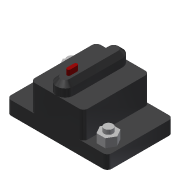
# Autodesk Inventor part: 120 Amp Breaker - Bussman
Saved by Autodesk Inventor 2013 (Build 170138000, 138)
## iProperties
Created: 2013-12-22
Part Number: 120 Amp Breaker - Bussman
Material: Generic
Document SubType Name: Modeling
Designer: Nemo
Mass: 108.862 g
Surface Area: 146.665 cm^2
Volume: 77.8352 cm^3
Density: 1.39862 g/cm^3
Author: Nemo
Autodesk Inventor part; units mm, degrees
ref_plane "YZ Plane" through (0, 0, 0) normal (1, 0, 0) x (0, 1, 0)
ref_plane "XZ Plane" through (0, 0, 0) normal (0, 1, 0) x (-1, 0, 0)
ref_plane "XY Plane" through (0, 0, 0) normal (0, 0, 1) x (1, 0, 0)
sketch "Sketch2" plane through (0, 0, 0) normal (0, 1, 0) x (-1, 0, 0)
  line L0 (36.83, -24.13) -> (-36.83, -24.13)
  line L1 (-36.83, -24.13) -> (-36.83, 24.13)
  line L2 (-36.83, 24.13) -> (36.83, 24.13)
  line L3 (36.83, 24.13) -> (36.83, -24.13)
  line L4 (36.83, -24.13) -> (-36.83, 24.13) construction
  line L5 (-36.83, -24.13) -> (36.83, 24.13) construction
  point P0 (0, 0)
  point P1 (0, 0)
  point P2 (0, 0)
  dimension "d2" = 73.66
  dimension "d3" = 48.26
  constraints: 12 end point, 3 midpoint, 2 parallel, 1 coincident, 1 horizontal, 1 perpendicular
  measures "d2" distance of L1.end L2.end
  measures "d3" distance of L0.end L1.end
extrude "Extrusion1" add sketch "Sketch2" along normal blind 9.906
sketch "Sketch3" plane through (0, 9.906, 0) normal (0, 1, 0) x (1, 0, 0)
  line L0 (36.83, 24.13) -> (-36.83, 24.13) projected
  line L1 (19.431, -24.13) -> (-19.431, -24.13)
  line L2 (-19.431, -24.13) -> (-19.431, 24.13)
  line L3 (-19.431, 24.13) -> (19.431, 24.13)
  line L4 (19.431, 24.13) -> (19.431, -24.13)
  line L5 (19.431, -24.13) -> (-19.431, 24.13) construction
  line L6 (-19.431, -24.13) -> (19.431, 24.13) construction
  point P0 (0, 0)
  dimension "d6" = 38.862
  constraints: 12 end point, 2 midpoint, 2 parallel, 1 horizontal, 1 perpendicular, 1 point on line
  measures "d6" distance of L2.end L3.end
extrude "Extrusion2" add sketch "Sketch3" along normal blind 19.5326
sketch "Sketch4" plane through (0, 29.4386, 0) normal (0, 1, 0) x (1, 0, 0)
  line L0 (19.431, 24.13) -> (-19.431, 24.13) projected
  line L1 (5.9238, -24.13) -> (-6.7762, -24.13)
  line L2 (-6.7762, -24.13) -> (-6.7762, 24.13)
  line L3 (-6.7762, 24.13) -> (5.9238, 24.13)
  line L4 (5.9238, 24.13) -> (5.9238, -24.13)
  line L5 (5.9238, -24.13) -> (-6.7762, 24.13) construction
  line L6 (-6.7762, -24.13) -> (5.9238, 24.13) construction
  line L7 (-19.431, -24.13) -> (19.431, -24.13) projected
  point P0 (0, 0)
  point P1 (-0.4262, 0)
  dimension "d9" = 12.7
  constraints: 12 end point, 2 midpoint, 2 parallel, 2 point on line, 1 horizontal, 1 perpendicular
  measures "d9" distance of L2.end L3.end
extrude "Extrusion3" add sketch "Sketch4" along normal blind 8.89
fillet "Fillet1" radius 6.35 4 edges at (-6.7762, 33.8836, 24.13) (5.9238, 33.8836, 24.13) (5.9238, 33.8836, -24.13) (-6.7762, 33.8836, -24.13)
chamfer "Chamfer1" distance 3.175 angle 45 4 edges at (-6.7762, 38.3286, 0) (-4.9164, 38.3286, 22.2702) (5.9238, 38.3286, 0) (4.0639, 38.3286, -22.2702)
sketch "Sketch5" plane through (0, 38.3286, 0) normal (0, 1, 0) x (1, 0, 0)
  arc A0 (-3.6012, -17.78) -> (2.7488, -17.78) centre (-0.4262, -17.78) ccw construction
  line L0 (-1.6327, -15.24) -> (0.9073, -15.24)
  line L1 (0.9073, -15.24) -> (0.9073, -10.16)
  line L2 (0.9073, -10.16) -> (-1.6327, -10.16)
  line L3 (-1.6327, -10.16) -> (-1.6327, -15.24)
  line L4 (-1.6327, -15.24) -> (0.9073, -10.16) construction
  line L5 (0.9073, -15.24) -> (-1.6327, -10.16) construction
  arc A1 (0.9073, -10.16) -> (-1.6327, -10.16) centre (-0.3627, -10.16) ccw
  arc A2 (-1.6327, -15.24) -> (0.9073, -15.24) centre (-0.3627, -15.24) ccw
  point P0 (0, 0)
  point P1 (-0.3627, -12.7)
  dimension "d16" = 5.08
  dimension "d18" = 2.54
  dimension "d19" = 2.54
  constraints: 12 end point, 4 point on circle, 4 tangent, 2 centre point, 2 midpoint, 2 parallel, 1 horizontal, 1 perpendicular
  measures "d16" distance between parallel lines of L0 L2
  measures "d18" distance of L1.end L2.end
  measures "d19" vertical distance of A0.centre A2.centre
extrude "Extrusion4" add sketch "Sketch5" along normal blind 3.81 separate body
sketch "Sketch6" plane through (0, 9.906, 0) normal (0, 1, 0) x (1, 0, 0)
  line L0 (19.431, -24.13) -> (36.83, -24.13) projected
  line L1 (-19.431, -24.13) -> (-19.431, 24.13) projected
  line L2 (-19.431, 24.13) -> (-36.83, 24.13) projected
  line L3 (-36.83, 24.13) -> (-36.83, -24.13) projected
  line L4 (-36.83, -24.13) -> (-19.431, -24.13) projected
  line L5 (-31.3384, 20.1613) -> (-24.9226, 20.1613)
  line L6 (-24.9226, 20.1613) -> (-21.7147, 14.605)
  line L7 (-21.7147, 14.605) -> (-24.9226, 9.0487)
  line L8 (-24.9226, 9.0487) -> (-31.3384, 9.0487)
  line L9 (-31.3384, 9.0487) -> (-34.5463, 14.605)
  line L10 (-34.5463, 14.605) -> (-31.3384, 20.1613)
  line L11 (24.9226, -9.0487) -> (31.3384, -9.0488)
  line L12 (31.3384, -9.0488) -> (34.5463, -14.605)
  line L13 (34.5463, -14.605) -> (31.3384, -20.1613)
  line L14 (31.3384, -20.1613) -> (24.9226, -20.1612)
  line L15 (24.9226, -20.1612) -> (21.7147, -14.605)
  line L16 (21.7147, -14.605) -> (24.9226, -9.0487)
  point P0 (0, 0)
  point P1 (-28.1305, 14.605)
  point P2 (-28.1305, 24.13)
  point P3 (28.1305, -14.605)
  point P4 (28.1305, -24.13)
  dimension "d22" = 11.1125
  dimension "d23" = 9.525
  dimension "d24" = 9.525
  dimension "d25" = 11.1125
  constraints: 24 end point, 2 horizontal, 2 midpoint, 2 vertical alignment, 26 other
  measures "d22" distance between parallel lines of L8 L5
  measures "d23" distance from line of L2 point (-28.13, 14.605)
  measures "d24" distance of point (28.13, -24.13) point (28.13, -14.605)
  measures "d25" distance between parallel lines of L14 L11
extrude "Extrusion5" add sketch "Sketch6" along normal blind 6.35 separate body contours L5 L6 L7 L8 L9 L10 | L11 L12 L13 L14 L15 L16
sketch "Sketch7" plane through (0, 16.256, 0) normal (0, 1, 0) x (1, 0, 0)
  line L0 (31.3384, -9.0488) -> (24.9226, -9.0487) projected
  line L1 (24.9226, -9.0487) -> (21.7147, -14.605) projected
  line L2 (21.7147, -14.605) -> (24.9226, -20.1612) projected
  line L3 (24.9226, -20.1612) -> (31.3384, -20.1613) projected
  line L4 (31.3384, -20.1613) -> (34.5463, -14.605) projected
  line L5 (34.5463, -14.605) -> (31.3384, -9.0488) projected
  circle A0 centre (-28.1305, 14.605) radius 3.175
  circle A1 centre (28.1305, -14.605) radius 3.175
  point P0 (0, 0)
  dimension "d28" = 6.35
  dimension "d29" = 6.35
  constraints: 2 centre point
  measures "d28" diameter of A0
  measures "d29" diameter of A1
extrude "Extrusion6" add sketch "Sketch7" along normal blind 3.175 contours A0 | A1 bodies 3
fillet "Fillet2" radius 3.175 8 edges at (-19.431, 19.6723, 24.13) (19.431, 19.6723, 24.13) (19.431, 19.6723, -24.13) (-19.431, 19.6723, -24.13) (-36.83, 4.953, 24.13) (36.83, 4.953, 24.13) (36.83, 4.953, -24.13) (-36.83, 4.953, -24.13)
body "Solid1"
body "Solid2"
body "Solid3"
